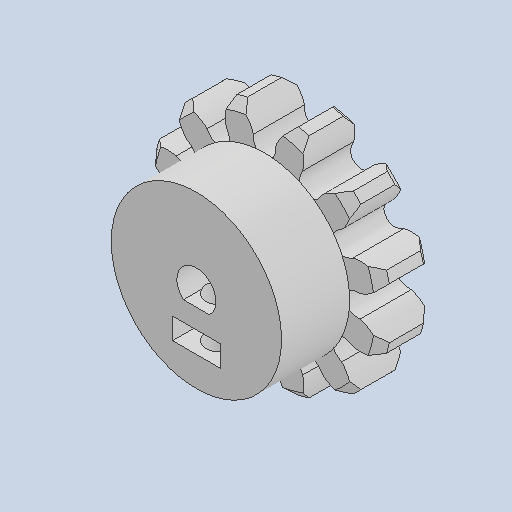
# Autodesk Inventor part: шестерня12_туу
Saved by Autodesk Inventor 2023.1 (Build 271208000, 208)
## iProperties
Created: 2025-10-14
Part Number: шестерня12_туу
Material: Generic
Document SubType Name: Modeling
Designer: DELL
Density: 1 g/cm^3
Appearance: Default
Author: DELL
Autodesk Inventor part; units mm, degrees
ref_plane "YZ Plane" through (0, 0, 0) normal (1, 0, 0) x (0, 1, 0)
ref_plane "XZ Plane" through (0, 0, 0) normal (0, 1, 0) x (-1, 0, 0)
ref_plane "XY Plane" through (0, 0, 0) normal (0, 0, 1) x (1, 0, 0)
sketch "Sketch1" plane through (0, 0, 0) normal (0, 0, 1) x (1, 0, 0)
  spline S0 degree 3 poles (-3.0087, 13.6604) (-2.9154, 13.5764) (-2.7289, 13.4085) (-2.4652, 13.1397) (-2.215, 12.8584) (-1.9815, 12.563) (-1.7672, 12.2533) (-1.608, 11.9827) (-1.4953, 11.7584) (-1.42, 11.586) (-1.3534, 11.4097) (-1.324, 11.2876) (-1.3093, 11.2266) knots 0 0 0 0 0.125009 0.250019 0.375027 0.500032 0.625031 0.750021 0.812526 0.87503 0.937528 1 1 1 1
  spline S1 degree 3 poles (-1.3093, 11.2266) (-1.3081, 11.1237) (-1.3062, 10.9693) (-1.2835, 10.7645) (-1.2555, 10.6127) (-1.2209, 10.4621) (-1.1712, 10.3158) (-1.1128, 10.1727) (-1.0388, 10.037) (-0.951, 9.9097) (-0.8483, 9.794) (-0.7312, 9.6929) (-0.6003, 9.6102) (-0.4585, 9.5481) (-0.3086, 9.5088) (-0.1543, 9.4971) (0, 9.5015) (0.1543, 9.4971) (0.3086, 9.5088) (0.4585, 9.5481) (0.6003, 9.6102) (0.7312, 9.6929) (0.8483, 9.794) (0.951, 9.9097) (1.0388, 10.037) (1.1128, 10.1727) (1.1712, 10.3158) (1.2209, 10.4621) (1.2555, 10.6127) (1.2835, 10.7645) (1.3062, 10.9693) (1.3081, 11.1237) (1.3093, 11.2266) knots 0 0 0 0 0.062509 0.093773 0.125034 0.156299 0.187559 0.218819 0.250082 0.281336 0.312585 0.343826 0.375061 0.406291 0.43751 0.468735 0.5 0.531265 0.56249 0.593709 0.624939 0.656174 0.687415 0.718664 0.749918 0.781181 0.812441 0.843701 0.874966 0.906227 0.937491 1 1 1 1
  spline S2 degree 3 poles (1.3093, 11.2266) (1.324, 11.2876) (1.3534, 11.4097) (1.42, 11.586) (1.4953, 11.7584) (1.608, 11.9827) (1.7672, 12.2533) (1.9815, 12.563) (2.215, 12.8584) (2.4652, 13.1397) (2.7289, 13.4085) (2.9154, 13.5764) (3.0087, 13.6604) knots 0 0 0 0 0.062472 0.12497 0.187474 0.249979 0.374969 0.499968 0.624973 0.749981 0.874991 1 1 1 1
  circle A0 centre (0, 0) radius 9.5 construction
  circle A1 centre (0, 0) radius 11.2763 construction
  circle A2 centre (0, 0) radius 12 construction
  circle A3 centre (0, 0) radius 13.9878
  point P0 (-2.7316, 13.4057)
  point P1 (-2.4675, 13.1376)
  point P2 (-2.2178, 12.856)
  point P3 (-1.9847, 12.5606)
  point P4 (-1.7711, 12.2508)
  point P5 (-1.5811, 11.926)
  point P6 (-1.4968, 11.7577)
  point P7 (-1.4215, 11.5853)
  point P8 (-1.3572, 11.4085)
  point P9 (-1.2988, 10.9182)
  point P10 (-1.2817, 10.7648)
  point P11 (-1.2544, 10.6129)
  point P12 (-1.2184, 10.4628)
  point P13 (-1.1698, 10.3163)
  point P14 (-1.1102, 10.1739)
  point P15 (-1.0365, 10.0384)
  point P16 (-0.9485, 9.9116)
  point P17 (-0.8459, 9.7964)
  point P18 (-0.7288, 9.6959)
  point P19 (-0.5984, 9.6136)
  point P20 (-0.4571, 9.5519)
  point P21 (-0.3079, 9.5134)
  point P22 (-0.1544, 9.4998)
  point P23 (0, 9.5)
  point P24 (0.1544, 9.4998)
  point P25 (0.3079, 9.5134)
  point P26 (0.4571, 9.5519)
  point P27 (0.5984, 9.6136)
  point P28 (0.7288, 9.6959)
  point P29 (0.8459, 9.7964)
  point P30 (0.9485, 9.9116)
  point P31 (1.0365, 10.0384)
  point P32 (1.1102, 10.1739)
  point P33 (1.1698, 10.3163)
  point P34 (1.2184, 10.4628)
  point P35 (1.2544, 10.6129)
  point P36 (1.2817, 10.7648)
  point P37 (1.2988, 10.9182)
  point P38 (1.3572, 11.4085)
  point P39 (1.4215, 11.5853)
  point P40 (1.4968, 11.7577)
  point P41 (1.5811, 11.926)
  point P42 (1.7711, 12.2508)
  point P43 (1.9847, 12.5606)
  point P44 (2.2178, 12.856)
  point P45 (2.4675, 13.1376)
  point P46 (2.7316, 13.4057)
  constraints: 4 centre point, 2 point on circle, 109 other
extrude "Выдавливание1" add sketch "Sketch1" against normal blind 6
extrude "Выдавливание2" cut sketch "Sketch1" against normal blind 10 contours A3 S2 S1 S0 picked at (-0.374, 12.578)
chamfer "Фаска1" distance 1 angle 45 2 edges at (0, -13.9878, 0) (0, -13.9878, -6)
pattern_circular "Круговой массив2" count 12 over 360 about axis through (0, 0, 0) along (0, 0, -1) of "Выдавливание2"
sketch "Эскиз2" plane through (0, 0, 0) normal (0, 0, 1) x (1, 0, 0)
  circle A0 centre (0, 0) radius 10
  dimension "d13" = 20
  constraints: 1 centre point, 1 coincident
  measures "d13" diameter of A0
extrude "Выдавливание3" add sketch "Эскиз2" along normal blind 8
sketch "Эскиз3" plane through (0, 0, 8) normal (0, 0, 1) x (1, 0, 0)
  arc A0 (1.5333, -1.7143) -> (-1.5333, -1.7143) centre (0, 0) ccw
  line L0 (1.5333, -1.7143) -> (-1.5333, -1.7143)
  dimension "d16" = 4.6
  constraints: 2 end point, 2 point on circle, 1 centre point, 1 coincident, 1 horizontal
  measures "d16" diameter of A0
extrude "Выдавливание4" cut sketch "Эскиз3" against normal blind 20
sketch "Эскиз4" plane through (0, 0, 8) normal (0, 0, 1) x (1, 0, 0)
  line L0 (-2.8, -4.0143) -> (2.8, -4.0143)
  line L1 (2.8, -4.0143) -> (2.8, -6.5143)
  line L2 (2.8, -6.5143) -> (-2.8, -6.5143)
  line L3 (-2.8, -6.5143) -> (-2.8, -4.0143)
  arc A0 (1.5333, -1.7143) -> (-1.5333, -1.7143) centre (0, 0) ccw projected
  line L4 (0, 0) -> (0, -9.2025) construction
  line L5 (1.5333, -1.7143) -> (-1.5333, -1.7143) projected
  point P0 (0, -4.0143)
  dimension "d23" = 5.6
  dimension "d24" = 2.5
  dimension "d25" = 2.3
  constraints: 10 end point, 2 parallel, 1 horizontal, 1 midpoint, 1 perpendicular, 1 point on line, 1 vertical
  measures "d23" distance of L1.end L2.end
  measures "d24" distance of L0.end L1.end
  measures "d25" distance between parallel lines of L5 L0
extrude "Выдавливание5" cut sketch "Эскиз4" against normal blind 6 contours L0 L1 L2 L3
sketch "Эскиз5" plane through (-2.8, -4.0143, 8) normal (0, -1, 0) x (1, 0, 0)
  circle A0 centre (2.8, -2.8) radius 1.65
  line L0 (4.3333, 0) -> (1.2667, 0) projected
  point P0 (2.8, -8)
  dimension "d28" = 3.3
  dimension "d32" = 5.2
  constraints: 1 centre point
  measures "d28" diameter of A0
  measures "d32" distance of point (2.8, -8) A0.centre
extrude "Выдавливание6" cut sketch "Эскиз5" along normal mid plane 13
equation "\"Модуль\" = 2"
equation "\"Угол_зацепления\" = 20deg"
equation "\"Зазор_профиля_зуба\" = 0.25"
equation "\"Радиус_закругления_зуба\" = 0.35"
equation "\"Диаметр_головки\" = 27.97554"
equation "\"Диаметр_впадин\" = 19"
equation "\"Основной_диаметр\" = 22.55262"
equation "\"Средний_диаметр\" = 24"
equation "\"Коэффициент_смещения\" = 0"
equation "\"Изменение_высоты_головки_зуба\" = 0.006115"
equation "\"Окружной_шаг\" = 6.283185"
equation "\"Общий_сдвиг_инструмента\" = 0"
equation "\"Внутренний\" = 0"
